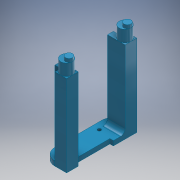
# Autodesk Inventor part: blue_part_modified
Saved by Autodesk Inventor 2017 SP1 (Build 210196100, 196)
## iProperties
Created: 2016-07-25
Part Number: blue_part_modified
Material: Plastique ABS
Document SubType Name: Modeling
Designer: tmonglon
Density: 1.06 g/cm^3
Appearance: Bleu ciel foncé
Author: tmonglon
Autodesk Inventor part; units mm, degrees
ref_plane "YZ Plane" through (0, 0, 0) normal (1, 0, 0) x (0, 1, 0)
ref_plane "XZ Plane" through (0, 0, 0) normal (0, 1, 0) x (-1, 0, 0)
ref_plane "XY Plane" through (0, 0, 0) normal (0, 0, 1) x (1, 0, 0)
sketch "Esquisse1" plane through (0, 0, 0) normal (0, 0, 1) x (1, 0, 0)
  line L0 (0, 0) -> (-10, 0)
  line L1 (-10, 0) -> (-10, 30)
  line L2 (-10, 30) -> (0, 30)
  line L3 (0, 0) -> (-5, 0)
  line L4 (-5, 0) -> (-5, 5)
  line L5 (-5, 5) -> (0, 5)
  line L6 (0, 5) -> (0, 0)
  line L7 (0, 4) -> (-3, 4)
  line L8 (-3, 4) -> (-3, 1)
  line L9 (-3, 1) -> (0, 1)
  line L10 (0, 1) -> (0, 4)
  line L11 (-1.5, 5) -> (-1.5, 20)
  line L12 (-1.5, 20) -> (0, 20)
  line L13 (0, 30) -> (0, 20)
  line L14 (0, 5) -> (0, 0)
  line L15 (0, 29) -> (-3, 29)
  line L16 (-3, 29) -> (-3, 26)
  line L17 (-3, 26) -> (0, 26)
  line L18 (0, 26) -> (0, 29)
  line L19 (0, 25) -> (-5, 25)
  line L20 (-5, 25) -> (-5, 30)
  line L21 (-5, 25) -> (-7.5, 25)
  line L22 (-7.5, 25) -> (-7.5, 27.5)
  line L23 (-7.5, 27.5) -> (-5, 27.5)
  line L24 (-5, 27.5) -> (-5, 25)
  line L25 (-5, 0) -> (-7.5, 0)
  line L26 (-5, 2.5) -> (-5, 0)
  line L27 (-5, 5) -> (-7.5, 5)
  line L28 (-7.5, 5) -> (-7.5, 2.5)
  line L29 (-7.5, 2.5) -> (-5, 2.5)
  line L30 (-5, 2.5) -> (-5, 5)
  line L31 (-3, 26) -> (0, 26)
  line L32 (0, 26) -> (0, 29)
  line L33 (0, 29) -> (-3, 29)
  line L34 (-3, 29) -> (-3, 26)
  line L35 (-3, 1) -> (0, 1)
  line L36 (0, 1) -> (0, 4)
  line L37 (0, 4) -> (-3, 4)
  line L38 (-3, 4) -> (-3, 1)
  dimension "d0" = 10
  dimension "d1" = 30
  dimension "d2" = 5
  dimension "d3" = 5
  dimension "d4" = 3
  dimension "d5" = 3
  dimension "d6" = 1
  dimension "d7" = 15
  dimension "d9" = 3
  dimension "d10" = 3
  dimension "d11" = 1
  dimension "d12" = 5
  dimension "d13" = 5
  dimension "d14" = 2.5
  dimension "d15" = 2.5
  dimension "d20" = 2.5
  dimension "d21" = 2.5
  constraints: 78 end point, 17 parallel, 11 perpendicular, 10 horizontal, 3 point on line, 2 midpoint, 1 vertical
  measures "d0" distance of L0.start L0.end
  measures "d1" distance of L2.end L0.start
  measures "d2" distance of L4.end L5.end
  measures "d3" distance of L3.end L4.end
  measures "d4" distance of L8.end L9.end
  measures "d5" distance of L7.end L8.end
  measures "d6" distance between parallel lines of L5 L7
  measures "d7" distance of L11.start L11.end
  measures "d9" distance of L15.end L16.end
  measures "d10" distance of L16.end L17.end
  measures "d11" distance between parallel lines of L2 L15
  measures "d12" distance of L19.start L19.end
  measures "d13" distance of L19.end L20.end
  measures "d14" distance of L22.end L23.end
  measures "d15" distance of L21.end L22.end
  measures "d20" distance of L28.end L29.end
  measures "d21" distance of L27.end L28.end
extrude "Extrusion1" add sketch "Esquisse1" along normal blind 40 contours L0 L4 L5 L6 L7 L8 L9 | L9 L8 L7 L6 | L2 L13 L15 L16 L17 L19 L20 | L13 L17 L16 L15
extrude "Extrusion2" add sketch "Esquisse1" along normal blind 35 contours L29 L28 L27 L4 | L20 L21 L22 L23
extrude "Extrusion3" add sketch "Esquisse1" along normal blind 41.5 contours L9 L8 L7 L6 | L13 L17 L16 L15
extrude "Extrusion4" add sketch "Esquisse1" along normal blind 2 contours L0 L1 L2 L20 L23 L22 L21 L19 L13 L12 L11 L5 L27 L28 L29 L4
fillet "Congé1" radius 5 2 edges at (-10, 0, 1) (-10, 30, 1)
sketch "Esquisse3" plane through (0, 0, 0) normal (0, 0, -1) x (-1, 0, 0)
  circle A0 centre (7, 9) radius 0.7
  circle A1 centre (7, 21) radius 0.7
  line L0 (0, 0) -> (0, 5) projected
  line L1 (0, 20) -> (0, 30) projected
  line L2 (5, 0) -> (0, 0) projected
  dimension "d29" = 1.4
  dimension "d30" = 1.4
  dimension "d31" = 12
  dimension "d32" = 7
  dimension "d33" = 7
  dimension "d34" = 9
  constraints: 2 centre point
  measures "d29" diameter of A0
  measures "d30" diameter of A1
  measures "d31" distance of A1.centre A0.centre
  measures "d32" distance from line of L0 A0.centre
  measures "d33" distance from line of L1 A1.centre
  measures "d34" distance from line of L2 A0.centre
extrude "Extrusion5" cut sketch "Esquisse3" against normal through all
fillet "Congé2" radius 2 2 edges at (-3.75, 25, 2) (-4.5, 5, 2)
sketch "Esquisse5" plane through (0, 0, 41.5) normal (0, 0, 1) x (1, 0, 0)
  line L0 (-3, 4) -> (0, 4) projected
  line L1 (0, 4) -> (0, 5) projected
  line L2 (0, 5) -> (-5, 5) projected
  line L3 (-5, 5) -> (-5, 0) projected
  line L4 (-5, 0) -> (0, 0) projected
  line L5 (0, 0) -> (0, 1) projected
  line L6 (0, 1) -> (-3, 1) projected
  line L7 (-3, 1) -> (-3, 4) projected
  line L8 (0, 1) -> (0, 4) projected
  line L9 (-3, 29) -> (0, 29) projected
  line L10 (0, 29) -> (0, 30) projected
  line L11 (0, 30) -> (-5, 30) projected
  line L12 (-5, 30) -> (-5, 25) projected
  line L13 (-5, 25) -> (0, 25) projected
  line L14 (0, 25) -> (0, 26) projected
  line L15 (0, 26) -> (-3, 26) projected
  line L16 (-3, 26) -> (-3, 29) projected
  line L17 (0, 26) -> (0, 29) projected
  line L18 (-5, 30) -> (-5, 25) projected
  circle A0 centre (-2.5, 27.5) radius 2.5
  circle A1 centre (-2.5, 2.5) radius 2.5
  circle A2 centre (-1.5, 27.5) radius 1.5
  circle A3 centre (-1.5, 2.5) radius 1.5
  constraints: 12 tangent, 4 centre point
extrude "Extrusion6" cut sketch "Esquisse5" against normal up to surface (1.5 mm away) contours L0 A3 L7 | L0 A1 A3 | A3 L6 L7 | L0 L8 A1 | L8 L6 A1 | A1 L6 A3 | L16 L15 A0 L9 | L9 A2 L16 | L9 A0 A2 | A2 L15 L16 | A0 L11 L10 L9 | L9 L17 A0 | L17 L15 A0 | A0 L15 A2 | A0 L12 L11 | L14 L13 A0 L15 | A0 L13 L12
sketch "Esquisse6" plane through (0, 0, 40) normal (0, 0, 1) x (1, 0, 0)
  circle A0 centre (-1.5, 27.5) radius 1.5 projected
  line L0 (0, 27.5) -> (0, 30) projected
  line L1 (0, 30) -> (-5, 30) projected
  line L2 (-5, 30) -> (-5, 25) projected
  line L3 (-5, 25) -> (0, 25) projected
  line L4 (0, 25) -> (0, 27.5) projected
  circle A1 centre (-1.5, 2.5) radius 1.5 projected
  line L5 (0, 2.5) -> (0, 5) projected
  line L6 (0, 5) -> (-5, 5) projected
  line L7 (-5, 5) -> (-5, 0) projected
  line L8 (-5, 0) -> (0, 0) projected
  line L9 (0, 0) -> (0, 2.5) projected
  circle A2 centre (-2.5, 2.5) radius 2.5
  circle A3 centre (-2.5, 27.5) radius 2.5
  constraints: 6 tangent, 2 centre point, 2 horizontal alignment
extrude "Extrusion7" cut sketch "Esquisse6" against normal up to surface (5 mm away) contours A3 L1 L0 | L4 L3 A3 | A3 L2 L1 | L3 L2 A3 | A2 L6 L5 | L9 L8 A2 | A2 L7 L6 | L8 L7 A2
